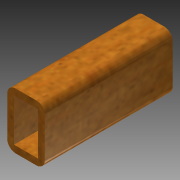
# Autodesk Inventor part: Sleeve
Saved by Autodesk Inventor 2015 (Build 190159000, 159)
## iProperties
Created: 2015-02-09
Part Number: Sleeve
Material: Generic
Document SubType Name: Modeling
Designer: paul
Density: 1 g/cm^3
Appearance: Default
Author: paul
Autodesk Inventor part; units mm, degrees
ref_plane "YZ Plane" through (0, 0, 0) normal (1, 0, 0) x (0, 1, 0)
ref_plane "XZ Plane" through (0, 0, 0) normal (0, 1, 0) x (-1, 0, 0)
sketch "Sketch1" plane through (0, 0, 0) normal (0, 0, 1) x (1, 0, 0)
  line L0 (-9, -8) -> (0, -8) projected
  line L1 (-9, -8) -> (-9, 8) projected
  line L2 (0, 8) -> (0, -8) projected
  line L3 (0, 8) -> (-9, 8) projected
  line L4 (-11.54, 10.54) -> (-11.54, -10.54)
  line L5 (-11.54, -10.54) -> (2.54, -10.54)
  line L6 (2.54, -10.54) -> (2.54, 10.54)
  line L7 (2.54, 10.54) -> (-11.54, 10.54)
  point P0 (0, 0)
  dimension "d0" = 2.54
  constraints: 8 end point, 3 other
  measures "d0" distance between parallel lines of L1 L4
ref_plane "Work Plane1" through (-9, -8, -48) normal (0, 0, -1) x (0, 1, 0)
extrude "Extrusion1" add sketch "Sketch1" against normal up to surface (48 mm away)
fillet "Fillet1" radius 3.175 4 edges at (-11.54, -10.54, -24) (2.54, -10.54, -24) (-11.54, 10.54, -24) (2.54, 10.54, -24)
body "Solid1"
